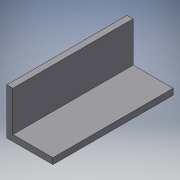
# Autodesk Inventor part: CameraLBracket
Saved by Autodesk Inventor 2019 (Build 230136000, 136)
## iProperties
Created: 2019-08-09
Part Number: CameraLBracket
Material: Generic
Document SubType Name: Modeling
Designer: aorfi
Density: 1 g/cm^3
Appearance: Default
Author: aorfi
Autodesk Inventor part; units mm, degrees
ref_plane "YZ Plane" through (0, 0, 0) normal (1, 0, 0) x (0, 1, 0)
ref_plane "XZ Plane" through (0, 0, 0) normal (0, 1, 0) x (-1, 0, 0)
ref_plane "XY Plane" through (0, 0, 0) normal (0, 0, 1) x (1, 0, 0)
sketch "Sketch1" plane through (0, 0, 0) normal (0, 1, 0) x (-1, 0, 0)
  line L0 (-11.5, 30) -> (11.5, 30)
  line L1 (11.5, 30) -> (11.5, -30)
  line L2 (11.5, -30) -> (-11.5, -30)
  line L3 (-11.5, -30) -> (-11.5, 30)
  line L4 (-11.5, 30) -> (11.5, -30) construction
  line L5 (11.5, 30) -> (-11.5, -30) construction
  point P0 (0, 0)
  dimension "d0" = 23
  dimension "d1" = 60
  constraints: 12 end point, 2 midpoint, 2 parallel, 1 horizontal, 1 perpendicular
  measures "d0" distance of L1.end L2.end
  measures "d1" distance of L0.end L1.end
extrude "Extrusion1" add sketch "Sketch1" along normal mid plane 3
sketch "Sketch2" plane through (0, 1.5, 0) normal (0, 1, 0) x (1, 0, 0)
  line L0 (-11.5, -30) -> (11.5, -30) projected
  line L1 (-11.5, -30) -> (-8.5, -30)
  line L2 (-8.5, -30) -> (-8.5, 30)
  line L3 (-8.5, 30) -> (-11.5, 30)
  line L4 (-11.5, 30) -> (-11.5, -30)
  line L5 (11.5, 30) -> (-11.5, 30) projected
  point P0 (0, 0)
  dimension "d4" = 3
  constraints: 8 end point, 2 parallel, 1 collinear, 1 horizontal, 1 perpendicular
  measures "d4" distance between parallel lines of L4 L2
extrude "Extrusion2" add sketch "Sketch2" along normal blind 20
body "Solid1"
